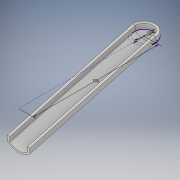
# Autodesk Inventor part: TOBOGAN
Saved by Autodesk Inventor 2019 (Build 230136000, 136)
## iProperties
Created: 2021-01-15
Part Number: TOBOGAN
Material: Générique
Document SubType Name: Modeling
Designer: tom.mousset
Density: 1 g/cm^3
Appearance: Par défaut
Author: tom.mousset
Autodesk Inventor part; units mm, degrees
ref_plane "YZ Plane" through (0, 0, 0) normal (1, 0, 0) x (0, 1, 0)
sketch "Esquisse1" plane through (0, 0, 0) normal (0, 1, 0) x (-1, 0, 0)
  line L0 (0, 0) -> (0, 100) construction
  circle A0 centre (0, 0) radius 7 construction
  circle A1 centre (0, 0) radius 9 construction
  arc A2 (-7, 0) -> (7, 0) centre (0, 0) ccw
  arc A3 (-9, 0) -> (9, 0) centre (0, 0) ccw
  line L1 (-9, 0) -> (-7, 0)
  line L2 (7, 0) -> (9, 0)
  line L3 (-7, 0) -> (-7, 2)
  line L4 (-7, 2) -> (-9, 2)
  line L5 (-9, 2) -> (-9, 0)
  line L6 (9, 0) -> (9, 2)
  line L7 (9, 2) -> (7, 2)
  line L8 (7, 2) -> (7, 0)
  dimension "d0" = 100
  dimension "d1" = 14
  dimension "d4" = 18
  dimension "d7" = 2
  constraints: 18 end point, 8 point on circle, 4 centre point, 4 coincident, 4 tangent, 3 perpendicular, 2 concentric, 2 equal length, 2 point on line, 2 vertical, 1 horizontal
  measures "d0" distance of L0.start L0.end
  measures "d1" diameter of A0
  measures "d4" diameter of A1
  measures "d7" distance of L1.end L3.end
ref_plane "Plan de construction1" through (9, -26.7949, 100) normal (1, 0, 0) x (0, 1, 0)
sketch "Esquisse3" plane through (9, -26.7949, 100) normal (1, 0, 0) x (0, 1, 0)
  line L0 (0, 0) -> (4, 0)
  line L1 (26.7949, -107) -> (26.7949, -100) projected
  line L2 (26.7949, -100) -> (30.7949, -100)
  line L3 (30.7949, -100) -> (4, 0)
  line L4 (26.7949, -100) -> (0, 0) projected
  line L5 (26.7949, -100) -> (0, 0)
  dimension "d12" = 4
  dimension "d13" = 4
  constraints: 8 end point, 2 horizontal, 1 collinear
  measures "d12" distance of L0.start L0.end
  measures "d13" distance of L1.end L2.end
extrude "Extrusion1" add sketch "Esquisse3" against normal blind 2
mirror "Symétrie1" about plane through (0, 0, 0) normal (1, 0, 0) of "Extrusion1"
ref_plane "Plan de construction2" through (7, 0, 0) normal (0, 1, 0) x (1, 0, 0)
sketch "Esquisse4" plane through (7, 0, 0) normal (0, 1, 0) x (1, 0, 0)
  arc A0 (2, 0) -> (-16, 0) centre (-7, 0) ccw projected
  arc A1 (2, 0) -> (-16, 0) centre (-7, 0) ccw
  arc A2 (0, 0) -> (-14, 0) centre (-7, 0) ccw projected
  arc A3 (0, 0) -> (-14, 0) centre (-7, 0) ccw
  line L0 (-14, -100) -> (-14, 0) projected
  line L1 (-14, 0) -> (-16, 0)
  line L2 (0, 0) -> (2, 0)
  constraints: 4 end point, 4 point on circle, 2 centre point, 2 coincident, 1 collinear, 1 perpendicular
extrude "Extrusion2" add sketch "Esquisse4" along normal blind 4
sketch "Esquisse5" plane through (9, -26.7949, 100) normal (0, 0, 1) x (1, 0, 0)
  line L0 (0, 0) -> (0, 26.7949) projected
  line L1 (-18, 0) -> (-18, 26.7949) projected
  line L2 (0, 0) -> (-18, 0)
  arc A0 (-18, 0) -> (0, 0) centre (-9, 9.3808) ccw
  line L3 (-16, 26.7949) -> (-16, 0) projected
  line L4 (-2, 26.7949) -> (-2, 0) projected
  arc A1 (-16, 0) -> (-2, 0) centre (-9, 9.3808) ccw
  point P0 (-9, 26.7949)
  dimension "d18" = 13
  constraints: 4 point on circle, 2 centre point, 2 end point, 1 concentric, 1 horizontal
  measures "d18" radius of A0
sketch3d "Esquisse 3D1"
  line L0 (9, -26.7949, 100) -> (9, 0, 0)
sweep "Balayage2" add profiles "Esquisse5" path "Esquisse 3D1" contours A0 L2 A1
sketch "Esquisse6" plane through (0, 0, 0) normal (0, 0, 1) x (1, 0, 0)
  arc A0 (-9, 0) -> (9, 0) centre (0, 9.3808) ccw projected
  line L0 (0, -3.6192) -> (0, -2.3239)
  arc A1 (-7, 0) -> (7, 0) centre (0, 9.3808) ccw projected
  line L1 (9, 0) -> (7, 0) projected
  line L2 (7, 0) -> (9, 0)
  line L3 (-7, 0) -> (7, 0) projected
  arc A2 (0, -2.3239) -> (7, 0) centre (0, 9.3808) ccw
  arc A3 (0, -3.6192) -> (9, 0) centre (0, 9.3808) ccw
  line L4 (0, -7.2643) -> (0, 12.155) projected
  point P0 (0, 0)
  constraints: 6 point on circle, 4 end point, 2 centre point, 1 collinear, 1 concentric, 1 vertical
revolve "Révolution1" add sketch "Esquisse6" angle 180 about axis through (0, -10, 0) along (0, 1, 0) contours L0 A1 L1 A0
